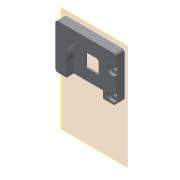
# Autodesk Inventor part: 30_cellSTORM_laserbase_ESP32cameradapter_v3
Saved by Autodesk Inventor 2019.4 (Build 234330000, 330)
## iProperties
Created: 2021-07-15
Part Number: 30_cellSTORM_laserbase_ESP32cameradapter_v3
Material: Generic
Document SubType Name: Modeling
Designer: diederichbenedict
Density: 1 g/cm^3
Appearance: Default
Author: diederichbenedict
Autodesk Inventor part; units mm, degrees
ref_plane "YZ Plane" through (0, 0, 0) normal (1, 0, 0) x (0, 1, 0)
ref_plane "XZ Plane" through (0, 0, 0) normal (0, 1, 0) x (-1, 0, 0)
ref_plane "XY Plane" through (0, 0, 0) normal (0, 0, 1) x (1, 0, 0)
ref_plane "Work Plane1" through (0, 0, 0) normal (0, 0, 1) x (1, 0, 0)
sketch "Sketch1" plane through (0, 0, 0) normal (0, 0, 1) x (1, 0, 0)
  line L0 (9.7547, 0) -> (-32, 0) construction
  line L1 (-32, 0) -> (-32, -5) construction
  line L2 (-5, -5) -> (-32, -5) construction
  line L3 (-5, -30.7015) -> (-5, -5) construction
  line L4 (-0.2453, -30.7015) -> (-5, -30.7015) construction
  line L5 (-0.2453, -30.7015) -> (-0.2453, -31) construction
  line L6 (-0.2453, -31) -> (4.1607, -31) construction
  line L7 (4.1607, -66) -> (4.1607, -31) projected
  line L8 (9.7547, -66) -> (4.1607, -66) projected
  line L9 (9.7547, 0) -> (9.7547, -66) projected
  circle A0 centre (-2.5, -10.3442) radius 1.45 construction
  circle A1 centre (-2.5, -25.9266) radius 1.45 construction
  circle A2 centre (-11.7453, -18.3978) radius 6 construction
  line L10 (-7.2453, -22.8978) -> (-16.2453, -22.8978)
  line L11 (-16.2453, -22.8978) -> (-16.2453, -13.8978)
  line L12 (-16.2453, -13.8978) -> (-7.2453, -13.8978)
  line L13 (-7.2453, -13.8978) -> (-7.2453, -22.8978)
  line L14 (-7.2453, -22.8978) -> (-16.2453, -13.8978)
  line L15 (-16.2453, -22.8978) -> (-7.2453, -13.8978)
  line L16 (9.7547, 0) -> (-32, 0) projected
  line L17 (9.7547, 0) -> (-32, 0) construction
  line L18 (-32, 0) -> (-32, -5) construction
  line L19 (-5, -5) -> (-32, -5) construction
  line L20 (-5, -30.7015) -> (-5, -5) construction
  line L21 (-0.2453, -30.7015) -> (-5, -30.7015) construction
  line L22 (-0.2453, -30.7015) -> (-0.2453, -31) construction
  line L23 (-0.2453, -31) -> (4.1607, -31) construction
  line L24 (4.1607, -66) -> (4.1607, -31) construction
  line L25 (9.7547, -66) -> (4.1607, -66) construction
  line L26 (9.7547, 0) -> (9.7547, -66) construction
  circle A3 centre (-2.5, -10.3442) radius 1.45 construction
  circle A4 centre (-2.5, -25.9266) radius 1.45 construction
  line L27 (9.7547, 0) -> (-32, 0)
  line L28 (-32, 0) -> (-32, -30.7015)
  line L29 (-32, -30.7015) -> (9.7547, -30.7015)
  line L30 (9.7547, -30.7015) -> (9.7547, 0)
  circle A5 centre (-2.5, -25.9266) radius 1.65
  circle A6 centre (-2.5, -10.3442) radius 1.65
  circle A7 centre (6.9577, -25.9266) radius 1.45 projected
  circle A8 centre (6.9577, -10.3442) radius 1.45 projected
  circle A9 centre (6.9577, -25.9266) radius 1.45 projected
  circle A10 centre (6.9577, -10.3442) radius 1.45 projected
  point P0 (0, 0)
  dimension "d0" = 9
  dimension "d1" = 9
  dimension "d2" = 3.3
  dimension "d3" = 3.3
  constraints: 20 end point, 4 parallel, 2 centre point, 2 coincident, 2 horizontal, 2 midpoint, 2 perpendicular
  measures "d0" distance of L11.end L12.end
  measures "d1" distance of L10.end L11.end
  measures "d2" diameter of A5
  measures "d3" diameter of A6
extrude "Extrusion1" add sketch "Sketch1" along normal blind 6 contours L9 L29 L28 L16 | A5 | A6 | A7 | A8
sketch "Sketch2" plane through (0, 0, 6) normal (0, 0, 1) x (1, 0, 0)
  circle A0 centre (-2.5, -25.9266) radius 1.65 projected
  circle A1 centre (-2.5, -10.3442) radius 1.65 projected
  circle A2 centre (6.9577, -25.9266) radius 1.45 projected
  circle A3 centre (6.9577, -10.3442) radius 1.45 projected
  point P0 (0, 0)
hole "Hole1" at (6.9577, -25.9266, 6) at (6.9577, -10.3442, 6) direction (0, 0, -1) diameter 3 end through all counterbore diameter 7 counterbore depth 2
fillet "Fillet1" radius 2 4 edges at (-32, 0, 3) (9.7547, 0, 3) (9.7547, -30.7015, 3) (-32, -30.7015, 3)
sketch "Sketch3" plane through (0, 0, 6) normal (0, 0, 1) x (1, 0, 0)
  line L0 (-16.2453, -22.8978) -> (-16.2453, -13.8978) projected
  line L1 (-7.2453, -13.8978) -> (-7.2453, -22.8978) projected
  line L2 (-7.2453, -22.8978) -> (-16.2453, -22.8978) projected
  circle A0 centre (-11.7453, -18.3978) radius 6 projected
  circle A1 centre (-11.7453, -18.3978) radius 12.75
  line L3 (-24.4953, -18.3978) -> (1.0047, -18.3978)
  line L4 (0.7547, -46.1354) -> (-24.2453, -46.1354)
  line L5 (-24.2453, -46.1354) -> (-24.2453, -20.9102)
  line L6 (-24.2453, -20.9102) -> (0.7547, -20.9102)
  line L7 (0.7547, -20.9102) -> (0.7547, -46.1354)
  line L8 (0.7547, -46.1354) -> (-24.2453, -20.9102) construction
  line L9 (-24.2453, -46.1354) -> (0.7547, -20.9102) construction
  point P0 (0, 0)
  point P1 (-11.7453, -33.5228)
  dimension "d14" = 25.5
  dimension "d17" = 25
  constraints: 14 end point, 3 point on circle, 2 horizontal, 2 midpoint, 2 parallel, 1 centre point, 1 coincident, 1 perpendicular
  measures "d14" diameter of A1
  measures "d17" distance between parallel lines of L7 L5
extrude "Extrusion2" cut sketch "Sketch3" against normal blind 5
sketch "Sketch4" plane through (0, 0, 6) normal (0, 0, 1) x (1, 0, 0)
  line L0 (0.7547, -20.9102) -> (0.7547, -30.7015) projected
  line L1 (0.7547, -30.7015) -> (7.7547, -30.7015) projected
  arc A0 (7.7547, -30.7015) -> (9.7547, -28.7015) centre (7.7547, -28.7015) ccw projected
  line L2 (9.7547, -28.7015) -> (9.7547, -28.0305) projected
  arc A1 (9.7547, -23.8226) -> (9.7547, -28.0305) centre (6.9577, -25.9266) ccw projected
  line L3 (9.7547, -23.8226) -> (9.7547, -12.4481) projected
  arc A2 (9.7547, -8.2402) -> (9.7547, -12.4481) centre (6.9577, -10.3442) ccw projected
  line L4 (9.7547, -8.2402) -> (9.7547, -2) projected
  arc A3 (9.7547, -2) -> (7.7547, 0) centre (7.7547, -2) ccw projected
  line L5 (7.7547, 0) -> (-30, 0) projected
  arc A4 (-30, 0) -> (-32, -2) centre (-30, -2) ccw projected
  line L6 (-32, -2) -> (-32, -28.7015) projected
  arc A5 (-32, -28.7015) -> (-30, -30.7015) centre (-30, -28.7015) ccw projected
  line L7 (-30, -30.7015) -> (-24.2453, -30.7015) projected
  line L8 (-24.2453, -30.7015) -> (-24.2453, -20.9102) projected
  arc A6 (0.7547, -20.9102) -> (-24.2453, -20.9102) centre (-11.7453, -18.3978) ccw projected
  line L9 (0.7547, -30.7015) -> (7.7547, -30.7015) projected
  line L10 (-24.2453, -30.7015) -> (0.7547, -30.7015)
  line L11 (-16.2453, -13.8978) -> (-16.2453, -22.8978) projected
  line L12 (-16.2453, -22.8978) -> (-7.2453, -22.8978) projected
  line L13 (-7.2453, -13.8978) -> (-16.2453, -13.8978) projected
  line L14 (-7.2453, -22.8978) -> (-7.2453, -13.8978) projected
  point P0 (0, 0)
  constraints: 2 end point, 1 collinear
extrude "Extrusion3" add sketch "Sketch4" along normal blind 3
sketch "Sketch5" plane through (0, 0, 9) normal (0, 0, 1) x (1, 0, 0)
  line L0 (-16.2453, -22.8978) -> (-16.2453, -13.8978) projected
  line L1 (-7.2453, -13.8978) -> (-7.2453, -22.8978) projected
  line L2 (-7.2453, -22.8978) -> (-16.2453, -22.8978) projected
  line L3 (-16.2453, -13.8978) -> (-7.2453, -13.8978) projected
  line L4 (-7.2453, -13.8978) -> (-7.2453, -22.8978) projected
  line L5 (-7.2453, -22.8978) -> (-16.2453, -22.8978) projected
  line L6 (-16.2453, -22.8978) -> (-16.2453, -13.8978) projected
  line L7 (-30, -30.7015) -> (7.7547, -30.7015) projected
  arc A0 (7.7547, -30.7015) -> (9.7547, -28.7015) centre (7.7547, -28.7015) ccw projected
  line L8 (9.7547, -28.7015) -> (9.7547, -28.0305) projected
  arc A1 (9.7547, -23.8226) -> (9.7547, -28.0305) centre (6.9577, -25.9266) ccw projected
  line L9 (9.7547, -23.8226) -> (9.7547, -12.4481) projected
  arc A2 (9.7547, -8.2402) -> (9.7547, -12.4481) centre (6.9577, -10.3442) ccw projected
  line L10 (9.7547, -8.2402) -> (9.7547, -2) projected
  arc A3 (9.7547, -2) -> (7.7547, 0) centre (7.7547, -2) ccw projected
  line L11 (7.7547, 0) -> (-30, 0) projected
  arc A4 (-30, 0) -> (-32, -2) centre (-30, -2) ccw projected
  line L12 (-32, -2) -> (-32, -28.7015) projected
  arc A5 (-32, -28.7015) -> (-30, -30.7015) centre (-30, -28.7015) ccw projected
  line L13 (-3.2453, -9.8978) -> (-20.2453, -9.8978)
  line L14 (-20.2453, -9.8978) -> (-20.2453, -26.8978)
  line L15 (-20.2453, -26.8978) -> (-3.2453, -26.8978)
  line L16 (-3.2453, -26.8978) -> (-3.2453, -9.8978)
  point P0 (0, 0)
  dimension "d20" = 4
  constraints: 8 end point, 3 other
  measures "d20" distance between parallel lines of L3 L13
extrude "Extrusion4" add sketch "Sketch5" along normal blind 45 contours L16 L15 L14 L13
fillet "Fillet2" radius 5 4 edges at (-3.2453, -26.8978, 31.5) (-20.2453, -26.8978, 31.5) (-3.2453, -9.8978, 31.5) (-20.2453, -9.8978, 31.5)
body "Solid1"
